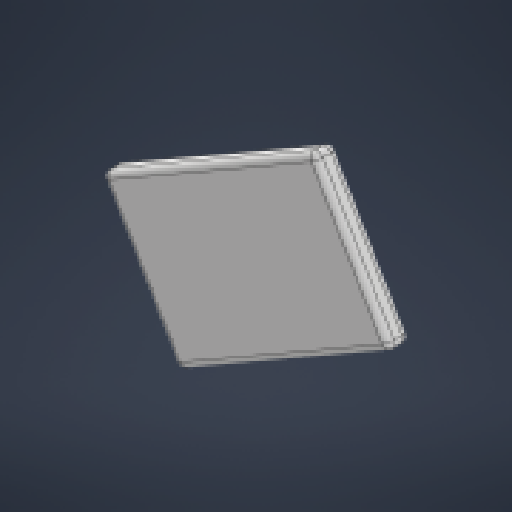
# Autodesk Inventor part: 503759
Saved by Autodesk Inventor 2023 (Build 270158000, 158)
## iProperties
Created: 2022-07-04
Part Number: 503759
Material: Generic
Document SubType Name: Modeling
Designer: jevan
Density: 1 g/cm^3
Appearance: Default
Author: jevan
Autodesk Inventor part; units mm, degrees
ref_plane "YZ Plane" through (0, 0, 0) normal (1, 0, 0) x (0, 1, 0)
ref_plane "XZ Plane" through (0, 0, 0) normal (0, 1, 0) x (-1, 0, 0)
ref_plane "XY Plane" through (0, 0, 0) normal (0, 0, 1) x (1, 0, 0)
sketch "Sketch1" plane through (0, 0, 0) normal (0, 0, 1) x (1, 0, 0)
  line L0 (0, 0) -> (25.5477, 14.75)
  line L1 (0, 0) -> (29.5, 0) construction
  line L2 (25.5477, 14.75) -> (16.2977, 30.7715)
  line L3 (-16.2977, -30.7715) -> (34.7977, -1.2715)
  line L4 (34.7977, -1.2715) -> (16.2977, 30.7715)
  line L5 (16.2977, 30.7715) -> (-34.7977, 1.2715)
  line L6 (-34.7977, 1.2715) -> (-16.2977, -30.7715)
  line L7 (-16.2977, -30.7715) -> (16.2977, 30.7715) construction
  line L8 (34.7977, -1.2715) -> (-34.7977, 1.2715) construction
  dimension "d0" = 29.5
  dimension "d1" = 30
  dimension "d2" = 18.5
  constraints: 18 end point, 3 parallel, 2 midpoint, 2 perpendicular, 1 equal length, 1 horizontal
  measures "d0" distance of L0.start L0.end
  measures "d1" angle of L1 L0
  measures "d2" distance of L0.end L2.end
extrude "Extrusion1" add sketch "Sketch1" along normal blind 5
fillet "Fillet1" radius 1.5 12 edges at (-9.25, 16.0215, 5) (-9.25, 16.0215, 0) (-34.7977, 1.2715, 2.5) (-25.5477, -14.75, 0) (-25.5477, -14.75, 5) (-16.2977, -30.7715, 2.5) (9.25, -16.0215, 5) (9.25, -16.0215, 0) (34.7977, -1.2715, 2.5) (20.9227, 22.7607, 0) (20.9227, 22.7607, 5) (16.2977, 30.7715, 2.5)
body "Solid1"
